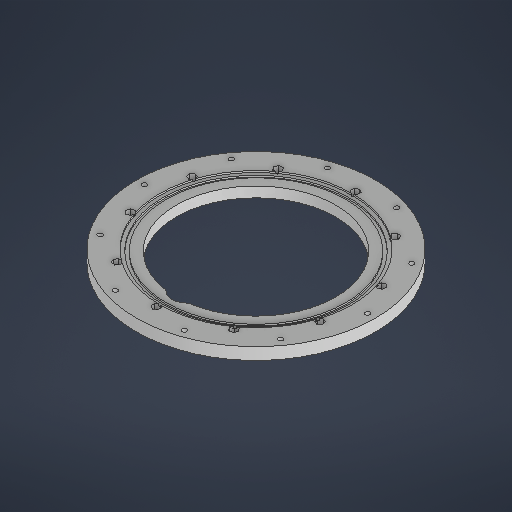
# Autodesk Inventor part: 260mm housing 2
Saved by Autodesk Inventor 2025 (Build 290162000, 162)
## iProperties
Created: 2024-10-30
Part Number: 260mm housing 2
Material: Generic
Document SubType Name: Modeling
Designer: mayhe
Density: 1 g/cm^3
Appearance: Default
Author: mayhe
Autodesk Inventor part; units mm, degrees
ref_plane "YZ Plane" through (0, 0, 0) normal (1, 0, 0) x (0, 1, 0)
sketch "Sketch1" plane through (0, 0, 0) normal (0, 1, 0) x (-1, 0, 0)
  circle A0 centre (0, 0) radius 150
  circle A1 centre (0, 0) radius 100
  circle A2 centre (0, 0) radius 125
  circle A3 centre (0, 125) radius 2.975
  line L0 (-4.375, 127.5259) -> (0, 130.0518)
  line L1 (0, 130.0518) -> (4.375, 127.5259)
  line L2 (4.375, 127.5259) -> (4.375, 122.4741)
  line L3 (4.375, 122.4741) -> (0, 119.9482)
  line L4 (0, 119.9482) -> (-4.375, 122.4741)
  line L5 (-4.375, 122.4741) -> (-4.375, 127.5259)
  circle A4 centre (-73.4732, 101.1271) radius 2.975
  line L6 (-78.4973, 100.5991) -> (-76.4425, 105.2141)
  line L7 (-76.4425, 105.2141) -> (-71.4184, 105.7422)
  line L8 (-71.4184, 105.7422) -> (-68.449, 101.6552)
  line L9 (-68.449, 101.6552) -> (-70.5038, 97.0401)
  line L10 (-70.5038, 97.0401) -> (-75.5279, 96.5121)
  line L11 (-75.5279, 96.5121) -> (-78.4973, 100.5991)
  circle A5 centre (-118.8821, 38.6271) radius 2.975
  line L12 (-122.6363, 35.2468) -> (-123.6866, 40.1882)
  line L13 (-123.6866, 40.1882) -> (-119.9324, 43.5685)
  line L14 (-119.9324, 43.5685) -> (-115.1278, 42.0074)
  line L15 (-115.1278, 42.0074) -> (-114.0775, 37.066)
  line L16 (-114.0775, 37.066) -> (-117.8317, 33.6857)
  line L17 (-117.8317, 33.6857) -> (-122.6363, 35.2468)
  circle A6 centre (-118.8821, -38.6271) radius 2.975
  line L18 (-119.9324, -43.5685) -> (-123.6866, -40.1882)
  line L19 (-123.6866, -40.1882) -> (-122.6363, -35.2468)
  line L20 (-122.6363, -35.2468) -> (-117.8317, -33.6857)
  line L21 (-117.8317, -33.6857) -> (-114.0775, -37.066)
  line L22 (-114.0775, -37.066) -> (-115.1278, -42.0074)
  line L23 (-115.1278, -42.0074) -> (-119.9324, -43.5685)
  circle A7 centre (-73.4732, -101.1271) radius 2.975
  line L24 (-71.4184, -105.7422) -> (-76.4425, -105.2141)
  line L25 (-76.4425, -105.2141) -> (-78.4973, -100.5991)
  line L26 (-78.4973, -100.5991) -> (-75.5279, -96.5121)
  line L27 (-75.5279, -96.5121) -> (-70.5038, -97.0401)
  line L28 (-70.5038, -97.0401) -> (-68.449, -101.6552)
  line L29 (-68.449, -101.6552) -> (-71.4184, -105.7422)
  circle A8 centre (0, -125) radius 2.975
  line L30 (4.375, -127.5259) -> (0, -130.0518)
  line L31 (0, -130.0518) -> (-4.375, -127.5259)
  line L32 (-4.375, -127.5259) -> (-4.375, -122.4741)
  line L33 (-4.375, -122.4741) -> (0, -119.9482)
  line L34 (0, -119.9482) -> (4.375, -122.4741)
  line L35 (4.375, -122.4741) -> (4.375, -127.5259)
  circle A9 centre (73.4732, -101.1271) radius 2.975
  line L36 (78.4973, -100.5991) -> (76.4425, -105.2141)
  line L37 (76.4425, -105.2141) -> (71.4184, -105.7422)
  line L38 (71.4184, -105.7422) -> (68.449, -101.6552)
  line L39 (68.449, -101.6552) -> (70.5038, -97.0401)
  line L40 (70.5038, -97.0401) -> (75.5279, -96.5121)
  line L41 (75.5279, -96.5121) -> (78.4973, -100.5991)
  circle A10 centre (118.8821, -38.6271) radius 2.975
  line L42 (122.6363, -35.2468) -> (123.6866, -40.1882)
  line L43 (123.6866, -40.1882) -> (119.9324, -43.5685)
  line L44 (119.9324, -43.5685) -> (115.1278, -42.0074)
  line L45 (115.1278, -42.0074) -> (114.0775, -37.066)
  line L46 (114.0775, -37.066) -> (117.8317, -33.6857)
  line L47 (117.8317, -33.6857) -> (122.6363, -35.2468)
  circle A11 centre (118.8821, 38.6271) radius 2.975
  line L48 (119.9324, 43.5685) -> (123.6866, 40.1882)
  line L49 (123.6866, 40.1882) -> (122.6363, 35.2468)
  line L50 (122.6363, 35.2468) -> (117.8317, 33.6857)
  line L51 (117.8317, 33.6857) -> (114.0775, 37.066)
  line L52 (114.0775, 37.066) -> (115.1278, 42.0074)
  line L53 (115.1278, 42.0074) -> (119.9324, 43.5685)
  circle A12 centre (73.4732, 101.1271) radius 2.975
  line L54 (71.4184, 105.7422) -> (76.4425, 105.2141)
  line L55 (76.4425, 105.2141) -> (78.4973, 100.5991)
  line L56 (78.4973, 100.5991) -> (75.5279, 96.5121)
  line L57 (75.5279, 96.5121) -> (70.5038, 97.0401)
  line L58 (70.5038, 97.0401) -> (68.449, 101.6552)
  line L59 (68.449, 101.6552) -> (71.4184, 105.7422)
  circle A13 centre (0, 125) radius 4.375
  point P0 (-4.375, 125)
  point P1 (-77.0126, 98.5556)
  point P2 (-120.234, 34.4663)
  point P3 (-117.5301, -42.788)
  point P4 (-69.9337, -103.6987)
  point P5 (4.375, -125)
  point P6 (77.0126, -98.5556)
  point P7 (120.234, -34.4663)
  point P8 (117.5301, 42.788)
  point P9 (69.9337, 103.6987)
  dimension "d2" = 250
  dimension "d0" = 300
  dimension "d1" = 200
  dimension "d7" = 5.95
  dimension "d11" = 360
  dimension "d64" = 8.75
  dimension "d65" = 125
  dimension "d66" = 125
  dimension "d67" = 8.75
  constraints: 120 end point, 13 centre point, 5 coincident, 1 midpoint, 1 tangent, 1 vertical alignment, 176 other
  measures "d0" diameter of A0
  measures "d1" diameter of A1
  measures "d7" diameter of A3
  measures "d64" diameter of A13
  measures "d65" distance of point (0, 0) A3.centre
  measures "d66" distance of point (0, 0) A13.centre
  measures "d67" distance between parallel lines of L0 L3
extrude "Extrusion1" add sketch "Sketch1" along normal blind 5 contours A0 | A2 L47 L46 L45 L44 L41 L40 L39 L38 L35 L34 L33 L32 L29 L28 L27 L26 L23 L22 L21 L20 L17 L16 L15 L14 L11 L10 L9 L8 L5 L4 L3 L2 L59 L58 L57 L56 L53 L52 L51 L50 | L50 L51 L52 L53 A2 A11 | A2 A11 L53 L48 L49 L50 | L47 L42 L43 L44 A2 A10 | A2 A10 L44 L45 L46 L47 | L56 L57 L58 L59 A2 A12 | A2 A12 L59 L54 L55 L56 | L41 L36 L37 L38 A2 A9 | A2 A9 L38 L39 L40 L41 | A13 A2 A3 | A2 A3 A13 L2 | L2 L3 A13 | L35 L30 L31 L32 A2 A8 | A2 A8 L32 L33 L34 L35 | A13 L1 L2 | L3 L4 A13 | A13 L0 L1 | L4 L5 A13 | L5 L0 A13 | L8 L9 L10 L11 A2 A4 | A2 A4 L11 L6 L7 L8 | L29 L24 L25 L26 A2 A7 | A2 A7 L26 L27 L28 L29 | L14 L15 L16 L17 A2 A5 | A2 A5 L17 L12 L13 L14 | L23 L18 L19 L20 A2 A6 | A2 A6 L20 L21 L22 L23
sketch "Sketch2" plane through (0, 5, 0) normal (0, 1, 0) x (1, 0, 0)
  point P0 (0, 0)
extrude "Extrusion2" add sketch "Sketch1" along normal blind 7.65 contours A0 | A2 L47 L46 L45 L44 L41 L40 L39 L38 L35 L34 L33 L32 L29 L28 L27 L26 L23 L22 L21 L20 L17 L16 L15 L14 L11 L10 L9 L8 L5 L4 L3 L2 L59 L58 L57 L56 L53 L52 L51 L50
sketch "Sketch3" plane through (0, 7.65, 0) normal (0, 1, 0) x (1, 0, 0)
  circle A0 centre (0, 0) radius 100
  circle A1 centre (0, 0) radius 150
  circle A2 centre (0, 125) radius 2.975 projected
  circle A3 centre (0, 0) radius 125
  circle A4 centre (0, 125) radius 2.975
  line L0 (-4.375, 127.5259) -> (0, 130.0518) projected
  line L1 (0, 130.0518) -> (4.375, 127.5259)
  line L2 (4.375, 127.5259) -> (4.375, 122.4741)
  line L3 (4.375, 122.4741) -> (0, 119.9482)
  line L4 (0, 119.9482) -> (-4.375, 122.4741)
  line L5 (-4.375, 122.4741) -> (-4.375, 127.5259)
  line L6 (-4.375, 127.5259) -> (0, 130.0518)
  circle A5 centre (-73.4732, 101.1271) radius 2.975
  line L7 (-76.4425, 105.2141) -> (-71.4184, 105.7422)
  line L8 (-71.4184, 105.7422) -> (-68.449, 101.6552)
  line L9 (-68.449, 101.6552) -> (-70.5038, 97.0401)
  line L10 (-70.5038, 97.0401) -> (-75.5279, 96.5121)
  line L11 (-75.5279, 96.5121) -> (-78.4973, 100.5991)
  line L12 (-78.4973, 100.5991) -> (-76.4425, 105.2141)
  circle A6 centre (-118.8821, 38.6271) radius 2.975
  line L13 (-123.6866, 40.1882) -> (-119.9324, 43.5685)
  line L14 (-119.9324, 43.5685) -> (-115.1278, 42.0074)
  line L15 (-115.1278, 42.0074) -> (-114.0775, 37.066)
  line L16 (-114.0775, 37.066) -> (-117.8317, 33.6857)
  line L17 (-117.8317, 33.6857) -> (-122.6363, 35.2468)
  line L18 (-122.6363, 35.2468) -> (-123.6866, 40.1882)
  circle A7 centre (-118.8821, -38.6271) radius 2.975
  line L19 (-123.6866, -40.1882) -> (-122.6363, -35.2468)
  line L20 (-122.6363, -35.2468) -> (-117.8317, -33.6857)
  line L21 (-117.8317, -33.6857) -> (-114.0775, -37.066)
  line L22 (-114.0775, -37.066) -> (-115.1278, -42.0074)
  line L23 (-115.1278, -42.0074) -> (-119.9324, -43.5685)
  line L24 (-119.9324, -43.5685) -> (-123.6866, -40.1882)
  circle A8 centre (-73.4732, -101.1271) radius 2.975
  line L25 (-76.4425, -105.2141) -> (-78.4973, -100.5991)
  line L26 (-78.4973, -100.5991) -> (-75.5279, -96.5121)
  line L27 (-75.5279, -96.5121) -> (-70.5038, -97.0401)
  line L28 (-70.5038, -97.0401) -> (-68.449, -101.6552)
  line L29 (-68.449, -101.6552) -> (-71.4184, -105.7422)
  line L30 (-71.4184, -105.7422) -> (-76.4425, -105.2141)
  circle A9 centre (0, -125) radius 2.975
  line L31 (0, -130.0518) -> (-4.375, -127.5259)
  line L32 (-4.375, -127.5259) -> (-4.375, -122.4741)
  line L33 (-4.375, -122.4741) -> (0, -119.9482)
  line L34 (0, -119.9482) -> (4.375, -122.4741)
  line L35 (4.375, -122.4741) -> (4.375, -127.5259)
  line L36 (4.375, -127.5259) -> (0, -130.0518)
  circle A10 centre (73.4732, -101.1271) radius 2.975
  line L37 (76.4425, -105.2141) -> (71.4184, -105.7422)
  line L38 (71.4184, -105.7422) -> (68.449, -101.6552)
  line L39 (68.449, -101.6552) -> (70.5038, -97.0401)
  line L40 (70.5038, -97.0401) -> (75.5279, -96.5121)
  line L41 (75.5279, -96.5121) -> (78.4973, -100.5991)
  line L42 (78.4973, -100.5991) -> (76.4425, -105.2141)
  circle A11 centre (118.8821, -38.6271) radius 2.975
  line L43 (123.6866, -40.1882) -> (119.9324, -43.5685)
  line L44 (119.9324, -43.5685) -> (115.1278, -42.0074)
  line L45 (115.1278, -42.0074) -> (114.0775, -37.066)
  line L46 (114.0775, -37.066) -> (117.8317, -33.6857)
  line L47 (117.8317, -33.6857) -> (122.6363, -35.2468)
  line L48 (122.6363, -35.2468) -> (123.6866, -40.1882)
  circle A12 centre (118.8821, 38.6271) radius 2.975
  line L49 (123.6866, 40.1882) -> (122.6363, 35.2468)
  line L50 (122.6363, 35.2468) -> (117.8317, 33.6857)
  line L51 (117.8317, 33.6857) -> (114.0775, 37.066)
  line L52 (114.0775, 37.066) -> (115.1278, 42.0074)
  line L53 (115.1278, 42.0074) -> (119.9324, 43.5685)
  line L54 (119.9324, 43.5685) -> (123.6866, 40.1882)
  circle A13 centre (73.4732, 101.1271) radius 2.975
  line L55 (76.4425, 105.2141) -> (78.4973, 100.5991)
  line L56 (78.4973, 100.5991) -> (75.5279, 96.5121)
  line L57 (75.5279, 96.5121) -> (70.5038, 97.0401)
  line L58 (70.5038, 97.0401) -> (68.449, 101.6552)
  line L59 (68.449, 101.6552) -> (71.4184, 105.7422)
  line L60 (71.4184, 105.7422) -> (76.4425, 105.2141)
  point P0 (-2.1875, 128.7889)
  point P1 (-77.4699, 102.9066)
  point P2 (-78.4973, 100.5991)
  point P3 (-76.4425, 105.2141)
  point P4 (-123.1615, 37.7175)
  point P5 (-122.6363, 35.2468)
  point P6 (-123.6866, 40.1882)
  point P7 (-121.8095, -41.8784)
  point P8 (-119.9324, -43.5685)
  point P9 (-123.6866, -40.1882)
  point P10 (-73.9305, -105.4782)
  point P11 (-71.4184, -105.7422)
  point P12 (-76.4425, -105.2141)
  point P13 (2.1875, -128.7889)
  point P14 (4.375, -127.5259)
  point P15 (0, -130.0518)
  point P16 (77.4699, -102.9066)
  point P17 (78.4973, -100.5991)
  point P18 (76.4425, -105.2141)
  point P19 (123.1615, -37.7175)
  point P20 (122.6363, -35.2468)
  point P21 (123.6866, -40.1882)
  point P22 (121.8095, 41.8784)
  point P23 (119.9324, 43.5685)
  point P24 (123.6866, 40.1882)
  point P25 (73.9305, 105.4782)
  point P26 (71.4184, 105.7422)
  point P27 (-4.375, 127.5259)
  point P28 (0, 130.0518)
  dimension "d15" = 250
  dimension "d72" = 360
  dimension "d78" = 200
  constraints: 120 end point, 23 coincident, 12 centre point, 2 midpoint, 1 concentric, 1 vertical alignment, 206 other
  measures "d78" diameter of A0
extrude "Extrusion3" add sketch "Sketch3" along normal blind 3.35 contours A1 | L5 L4 L3 L2 A3 L59 L58 L57 L56 L53 L52 L51 L50 L47 L46 L45 L44 L41 L40 L39 L38 L35 L34 L33 L32 L29 L28 L27 L26 L23 L22 L21 L20 L17 L16 L15 L14 L11 L10 L9 L8
sketch "Sketch5" plane through (0, 11, 0) normal (0, 1, 0) x (1, 0, 0)
  circle A0 centre (0, 0) radius 100
  circle A1 centre (0, 0) radius 150
  circle A2 centre (0, 125) radius 2.975 projected
  line L0 (-4.375, 127.5259) -> (0, 130.0518) projected
  line L1 (0, 130.0518) -> (4.375, 127.5259)
  line L2 (4.375, 127.5259) -> (4.375, 122.4741)
  line L3 (4.375, 122.4741) -> (0, 119.9482)
  line L4 (0, 119.9482) -> (-4.375, 122.4741)
  line L5 (-4.375, 122.4741) -> (-4.375, 127.5259)
  line L6 (-4.375, 127.5259) -> (0, 130.0518)
  circle A3 centre (0, 0) radius 125
  line L7 (-76.4425, 105.2141) -> (-71.4184, 105.7422)
  line L8 (-71.4184, 105.7422) -> (-68.449, 101.6552)
  line L9 (-68.449, 101.6552) -> (-70.5038, 97.0401)
  line L10 (-70.5038, 97.0401) -> (-75.5279, 96.5121)
  line L11 (-75.5279, 96.5121) -> (-78.4973, 100.5991)
  line L12 (-78.4973, 100.5991) -> (-76.4425, 105.2141)
  line L13 (-123.6866, 40.1882) -> (-119.9324, 43.5685)
  line L14 (-119.9324, 43.5685) -> (-115.1278, 42.0074)
  line L15 (-115.1278, 42.0074) -> (-114.0775, 37.066)
  line L16 (-114.0775, 37.066) -> (-117.8317, 33.6857)
  line L17 (-117.8317, 33.6857) -> (-122.6363, 35.2468)
  line L18 (-122.6363, 35.2468) -> (-123.6866, 40.1882)
  line L19 (-123.6866, -40.1882) -> (-122.6363, -35.2468)
  line L20 (-122.6363, -35.2468) -> (-117.8317, -33.6857)
  line L21 (-117.8317, -33.6857) -> (-114.0775, -37.066)
  line L22 (-114.0775, -37.066) -> (-115.1278, -42.0074)
  line L23 (-115.1278, -42.0074) -> (-119.9324, -43.5685)
  line L24 (-119.9324, -43.5685) -> (-123.6866, -40.1882)
  line L25 (-76.4425, -105.2141) -> (-78.4973, -100.5991)
  line L26 (-78.4973, -100.5991) -> (-75.5279, -96.5121)
  line L27 (-75.5279, -96.5121) -> (-70.5038, -97.0401)
  line L28 (-70.5038, -97.0401) -> (-68.449, -101.6552)
  line L29 (-68.449, -101.6552) -> (-71.4184, -105.7422)
  line L30 (-71.4184, -105.7422) -> (-76.4425, -105.2141)
  line L31 (0, -130.0518) -> (-4.375, -127.5259)
  line L32 (-4.375, -127.5259) -> (-4.375, -122.4741)
  line L33 (-4.375, -122.4741) -> (0, -119.9482)
  line L34 (0, -119.9482) -> (4.375, -122.4741)
  line L35 (4.375, -122.4741) -> (4.375, -127.5259)
  line L36 (4.375, -127.5259) -> (0, -130.0518)
  line L37 (76.4425, -105.2141) -> (71.4184, -105.7422)
  line L38 (71.4184, -105.7422) -> (68.449, -101.6552)
  line L39 (68.449, -101.6552) -> (70.5038, -97.0401)
  line L40 (70.5038, -97.0401) -> (75.5279, -96.5121)
  line L41 (75.5279, -96.5121) -> (78.4973, -100.5991)
  line L42 (78.4973, -100.5991) -> (76.4425, -105.2141)
  line L43 (123.6866, -40.1882) -> (119.9324, -43.5685)
  line L44 (119.9324, -43.5685) -> (115.1278, -42.0074)
  line L45 (115.1278, -42.0074) -> (114.0775, -37.066)
  line L46 (114.0775, -37.066) -> (117.8317, -33.6857)
  line L47 (117.8317, -33.6857) -> (122.6363, -35.2468)
  line L48 (122.6363, -35.2468) -> (123.6866, -40.1882)
  line L49 (123.6866, 40.1882) -> (122.6363, 35.2468)
  line L50 (122.6363, 35.2468) -> (117.8317, 33.6857)
  line L51 (117.8317, 33.6857) -> (114.0775, 37.066)
  line L52 (114.0775, 37.066) -> (115.1278, 42.0074)
  line L53 (115.1278, 42.0074) -> (119.9324, 43.5685)
  line L54 (119.9324, 43.5685) -> (123.6866, 40.1882)
  line L55 (76.4425, 105.2141) -> (78.4973, 100.5991)
  line L56 (78.4973, 100.5991) -> (75.5279, 96.5121)
  line L57 (75.5279, 96.5121) -> (70.5038, 97.0401)
  line L58 (70.5038, 97.0401) -> (68.449, 101.6552)
  line L59 (68.449, 101.6552) -> (71.4184, 105.7422)
  line L60 (71.4184, 105.7422) -> (76.4425, 105.2141)
  point P0 (-2.1875, 128.7889)
  point P1 (-73.4732, 101.1271)
  point P2 (-77.4699, 102.9066)
  point P3 (-118.8821, 38.6271)
  point P4 (-123.1615, 37.7175)
  point P5 (-118.8821, -38.6271)
  point P6 (-121.8095, -41.8784)
  point P7 (-73.4732, -101.1271)
  point P8 (-73.9305, -105.4782)
  point P9 (0, -125)
  point P10 (2.1875, -128.7889)
  point P11 (73.4732, -101.1271)
  point P12 (77.4699, -102.9066)
  point P13 (118.8821, -38.6271)
  point P14 (123.1615, -37.7175)
  point P15 (118.8821, 38.6271)
  point P16 (121.8095, 41.8784)
  point P17 (73.4732, 101.1271)
  point P18 (73.9305, 105.4782)
  point P19 (-4.375, 127.5259)
  point P20 (0, 130.0518)
  dimension "d76" = 360
  dimension "d79" = 200
  constraints: 120 end point, 4 coincident, 2 centre point, 2 midpoint, 1 vertical alignment, 156 other
  measures "d79" diameter of A0
extrude "Extrusion6" add sketch "Sketch5" along normal blind 4 contours A1 | L5 L4 L3 L2 A3 L59 L58 L57 L56 L53 L52 L51 L50 L47 L46 L45 L44 L41 L40 L39 L38 L35 L34 L33 L32 L29 L28 L27 L26 L23 L22 L21 L20 L17 L16 L15 L14 L11 L10 L9 L8
sketch "Sketch6" plane through (0, 15, 0) normal (0, 1, 0) x (1, 0, 0)
  circle A0 centre (0, 0) radius 120.75
  dimension "d29" = 241.5
  constraints: 1 centre point, 1 coincident
  measures "d29" diameter of A0
extrude "Extrusion7" cut sketch "Sketch6" against normal blind 2.125
sketch "Sketch8" plane through (0, 0, 0) normal (0, -1, 0) x (1, 0, 0)
  circle A0 centre (0, 0) radius 140
  circle A1 centre (140, 0) radius 2.75
  circle A2 centre (113.2624, 82.2899) radius 2.75
  circle A3 centre (43.2624, 133.1479) radius 2.75
  circle A4 centre (-43.2624, 133.1479) radius 2.75
  circle A5 centre (-113.2624, 82.2899) radius 2.75
  circle A6 centre (-140, 0) radius 2.75
  circle A7 centre (-113.2624, -82.2899) radius 2.75
  circle A8 centre (-43.2624, -133.1479) radius 2.75
  circle A9 centre (43.2624, -133.1479) radius 2.75
  circle A10 centre (113.2624, -82.2899) radius 2.75
  dimension "d45" = 280
  dimension "d46" = 5.5
  dimension "d49" = 360
  constraints: 10 centre point, 1 coincident, 1 horizontal alignment, 23 other
  measures "d46" diameter of A1
hole "Hole2" at (-43.2624, 0, -133.1479) at (-113.2624, 0, -82.2899) at (-140, 0, 0) at (-113.2624, 0, 82.2899) at (-43.2624, 0, 133.1479) at (43.2624, 0, 133.1479) at (113.2624, 0, 82.2899) at (140, 0, 0) at (113.2624, 0, -82.2899) at (43.2624, 0, -133.1479) direction (0, 1, 0) diameter 5.95 end through all counterbore diameter 10.475 counterbore depth 7.375
sketch "Sketch9" plane through (0, 0, 0) normal (1, 0, 0) x (0, 1, 0)
  line L0 (12.875, -100) -> (12.875, 100) projected
  line L1 (12.875, -100) -> (-3.3103, -100)
  line L2 (12.875, -100) -> (0, -100) projected
  line L3 (14.875, -116.5) -> (10.875, -116.5)
  line L4 (10.875, -116.5) -> (10.875, -112.5)
  line L5 (10.875, -112.5) -> (14.875, -112.5)
  line L6 (14.875, -112.5) -> (14.875, -116.5)
  line L7 (12.875, 96.8741) -> (12.875, 38.6193) projected
  line L8 (14.875, -116.5) -> (10.875, -112.5) construction
  line L9 (10.875, -116.5) -> (14.875, -112.5) construction
  line L10 (2, -116.5) -> (-2, -116.5)
  line L11 (-2, -116.5) -> (-2, -112.5)
  line L12 (-2, -112.5) -> (2, -112.5)
  line L13 (2, -112.5) -> (2, -116.5)
  line L14 (0, -150) -> (0, 150) projected
  line L15 (2, -116.5) -> (-2, -112.5) construction
  line L16 (-2, -116.5) -> (2, -112.5) construction
  line L17 (-6.9474, 0) -> (18.5121, 0) projected
  point P0 (0, 0)
  point P1 (12.875, -114.5)
  point P2 (0, -114.5)
  dimension "d58" = 4
  dimension "d59" = 4
  dimension "d60" = 14.5
  dimension "d61" = 4
  dimension "d62" = 4
  constraints: 26 end point, 4 midpoint, 4 parallel, 2 horizontal, 2 perpendicular, 2 point on line, 2 other
  measures "d58" distance of L4.end L5.end
  measures "d59" distance of L3.end L4.end
  measures "d60" distance from line of L1 point (12.875, -114.5)
  measures "d61" distance of L11.end L12.end
  measures "d62" distance of L10.end L11.end
revolve "Revolution1" cut sketch "Sketch9" angle 360 about axis through (0, -10, 0) along (0, 1, 0) contours L12 L13 L10 L14 | L14 L10 L11 L12 | L3 L4 L5 L6
ref_plane "Work Plane3" through (7.9375, -10, 150.8125) normal (0, 0.9188, -0.3947) x (-1, 0, 0)
ref_plane "Work Plane4" through (7.9375, 48.3432, 125.7463) normal (0, 0.9188, -0.3947) x (-1, 0, 0)
sketch "Sketch13" plane through (7.9375, 48.3432, 125.7463) normal (0, 0.9188, -0.3947) x (-1, 0, 0)
  circle A0 centre (7.9375, -52.7148) radius 20
  point P0 (7.9375, -134.6178)
  dimension "d92" = 40
  dimension "d93" = 81.903
  constraints: 1 centre point
  measures "d92" diameter of A0
  measures "d93" distance of A0.centre point (7.938, -134.618)
extrude "Extrusion12" cut sketch "Sketch13" against normal blind 256.0625
body "Solid1"
